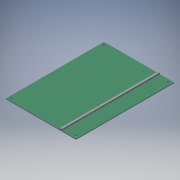
# Autodesk Inventor part: MockPCB
Saved by Autodesk Inventor 2017 (Build 210142000, 142)
## iProperties
Created: 2017-03-02
Part Number: MockPCB
Material: Generic
Document SubType Name: Modeling
Designer: hoeflinc
Density: 1 g/cm^3
Appearance: Default
Quantity: 1
Author: hoeflinc
Autodesk Inventor part; units mm, degrees
ref_plane "YZ Plane" through (0, 0, 0) normal (1, 0, 0) x (0, 1, 0)
ref_plane "XZ Plane" through (0, 0, 0) normal (0, 1, 0) x (-1, 0, 0)
ref_plane "XY Plane" through (0, 0, 0) normal (0, 0, 1) x (1, 0, 0)
sketch "Sketch1" plane through (0, 0, 0) normal (0, 1, 0) x (-1, 0, 0)
  line L0 (0, 0) -> (127, 0)
  line L1 (127, 0) -> (127, -177.8)
  line L2 (127, -177.8) -> (0, -177.8)
  line L3 (0, -177.8) -> (0, 0)
  dimension "d0" = 127
  dimension "d1" = 177.8
  constraints: 8 end point, 2 parallel, 1 horizontal, 1 perpendicular
  measures "d0" distance of L0.start L0.end
  measures "d1" distance of L2.end L0.start
extrude "Extrusion1" add sketch "Sketch1" along normal blind 1.5875
sketch "Sketch2" plane through (0, 1.5875, 0) normal (0, 1, 0) x (1, 0, 0)
  line L0 (-127, 177.8) -> (-127, 0) projected
  line L1 (0, 177.8) -> (-127, 177.8) projected
  line L2 (0, 0) -> (0, 177.8) projected
  line L3 (-127, 0) -> (0, 0) projected
  point P0 (-121.92, 172.72)
  point P1 (-5.08, 172.72)
  point P2 (-5.08, 5.08)
  point P3 (-121.92, 5.08)
  dimension "d4" = 5.08
  dimension "d5" = 5.08
  dimension "d6" = 5.08
  dimension "d7" = 5.08
  dimension "d8" = 5.08
  dimension "d9" = 5.08
  dimension "d10" = 5.08
  dimension "d11" = 5.08
  measures "d4" distance from line of L0 point (-121.92, 172.72)
  measures "d5" distance from line of L1 point (-121.92, 172.72)
  measures "d6" distance from line of L1 point (-5.08, 172.72)
  measures "d7" distance from line of L2 point (-5.08, 172.72)
  measures "d8" distance from line of L2 point (-5.08, 5.08)
  measures "d9" distance from line of point (-5.08, 5.08) L3
  measures "d10" distance from line of L3 point (-121.92, 5.08)
  measures "d11" distance from line of L0 point (-121.92, 5.08)
hole "Hole1" at (-121.92, 1.5875, -172.72) at (-5.08, 1.5875, -172.72) at (-5.08, 1.5875, -5.08) at (-121.92, 1.5875, -5.08) direction (0, -1, 0) diameter 3.5 end through all
sketch "Sketch3" plane through (0, 1.5875, 0) normal (0, 1, 0) x (1, 0, 0)
  circle A0 centre (-5.08, 5.08) radius 1.75 projected
  circle A1 centre (-121.92, 172.72) radius 1.75 projected
  circle A2 centre (-5.08, 172.72) radius 1.75 projected
  circle A3 centre (-121.92, 5.08) radius 1.75 projected
  line L0 (-127, 0) -> (0, 0) projected
  line L1 (0, 0) -> (0, 177.8) projected
  line L2 (0, 177.8) -> (-127, 177.8) projected
  line L3 (-127, 177.8) -> (-127, 0) projected
  line L4 (-127, 0) -> (0, 0) projected
  line L5 (0, 177.8) -> (-127, 177.8) projected
  line L6 (-28.9, 0) -> (-25.4, 0)
  line L7 (-25.4, 0) -> (-25.4, 177.8)
  line L8 (-25.4, 177.8) -> (-28.9, 177.8)
  line L9 (-28.9, 177.8) -> (-28.9, 0)
  dimension "d19" = 3.5
  dimension "d23" = 25.4
  constraints: 8 end point, 2 parallel, 2 point on line, 1 horizontal, 1 perpendicular
  measures "d19" distance between parallel lines of L7 L9
  measures "d23" distance between parallel lines of L7 L1
extrude "Extrusion2" add sketch "Sketch3" along normal blind 2.54 contours L9 L2 L7 L0
body "Solid1"
